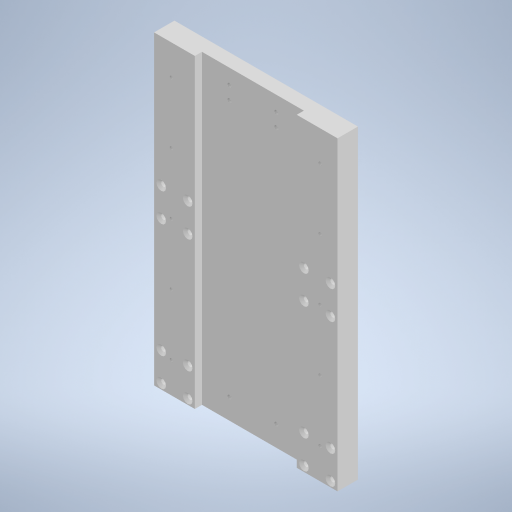
# Autodesk Inventor part: KreuzplatteNeu
Saved by Autodesk Inventor 2024 (Build 280153020, 153B)
## iProperties
Created: 2023-07-13
Part Number: KreuzplatteNeu
Material: Generisch
Document SubType Name: Modeling
Designer: hol
Density: 1 g/cm^3
Appearance: Vorgabe
Author: hol
Autodesk Inventor part; units mm, degrees
ref_plane "YZ Plane" through (0, 0, 0) normal (1, 0, 0) x (0, 1, 0)
ref_plane "XZ Plane" through (0, 0, 0) normal (0, 1, 0) x (-1, 0, 0)
ref_plane "XY Plane" through (0, 0, 0) normal (0, 0, 1) x (1, 0, 0)
sketch "Skizze1" plane through (0, 0, 0) normal (0, 1, 0) x (-1, 0, 0)
  line L0 (0, 0) -> (180, 0)
  line L1 (180, 0) -> (180, 300)
  line L2 (180, 300) -> (0, 300)
  line L3 (0, 300) -> (0, 0)
  dimension "Breite" = 180
  dimension "Höhe" = 300
  constraints: 8 end point, 2 parallel, 1 horizontal, 1 perpendicular
  measures "Breite" distance of L2.end L1.end
  measures "Höhe" distance of L1.end L0.end
extrude "Extrusion1" add sketch "Skizze1" along normal blind 20
sketch "Skizze2" plane through (0, 0, 0) normal (0, -1, 0) x (1, 0, 0)
  line L0 (-180, 300) -> (0, 300) projected
  line L1 (0, 300) -> (0, 0) projected
  line L2 (0, 0) -> (-180, 0) projected
  line L3 (-140, 300) -> (-40, 300)
  line L4 (-40, 300) -> (-40, 0)
  line L5 (-40, 0) -> (-140, 0)
  line L6 (-140, 0) -> (-140, 300)
  point P0 (-90, 300)
  point P1 (-140, 0)
  point P2 (-40, 300)
  dimension "d4" = 100
  constraints: 8 end point, 2 midpoint, 2 parallel, 2 point on line, 1 horizontal, 1 perpendicular
  measures "d4" distance of L3.start L3.end
extrude "Extrusion2" cut sketch "Skizze2" against normal blind 7 contours L0 L4 L2 L6
sketch "Skizze3" plane through (0, 0, 0) normal (0, -1, 0) x (1, 0, 0)
  line L0 (-180, 0) -> (-180, 300) projected
  line L1 (-140, 0) -> (-180, 0) projected
  line L2 (-40, 0) -> (-140, 0) projected
  line L3 (-173, 33.5) -> (-147, 33.5) construction
  line L4 (-147, 33.5) -> (-147, 5.5) construction
  line L5 (-147, 5.5) -> (-173, 5.5) construction
  line L6 (-173, 5.5) -> (-173, 33.5) construction
  point P0 (0, 0)
  dimension "SenkerY" = 26
  dimension "SenkerZ" = 28
  dimension "d9" = 7
  dimension "d10" = 5.5
  constraints: 8 end point, 4 coincident, 2 parallel, 1 horizontal, 1 perpendicular
  measures "SenkerY" distance of L3.start L3.end
  measures "SenkerZ" distance of L5.end L3.start
  measures "d9" distance from line of L0 L5.end
  measures "d10" distance between parallel lines of L1 L5
hole "Bohrung1" at (-173, 0, 5.5) at (-173, 0, 33.5) at (-147, 0, 33.5) at (-147, 0, 5.5) direction (0, 1, 0) diameter 4.8 depth 20 tip angle 118 countersink diameter 9.4 countersink angle 90 clearance for "Flachkopfsenkschraube ISO 2009/7046" size "M4" standard "ISO"
pattern_linear "Rechteckige Anordnung1" count 2 spacing 140 along (0, 0, 1) count 2 spacing 140 along (1, 0, 0) of "Bohrung1"
sketch "Skizze4" plane through (0, 0, 0) normal (0, -1, 0) x (1, 0, 0)
  line L0 (-180, 0) -> (-180, 300) projected
  line L1 (-180, 300) -> (0, 300) construction
  line L2 (-140, 0) -> (-180, 0) construction
  point P0 (0, 0)
  point P1 (-163, 30)
  point P2 (-160, 0)
  dimension "d25" = 30
  dimension "GleitschieneY" = 17
  constraints: 1 midpoint
  measures "d25" vertical distance of point (-160, 0) point (-163, 30)
  measures "GleitschieneY" distance from line of L0 point (-163, 30)
hole "Bohrung2" at (-163, 0, 30) direction (0, 1, 0) diameter 3.242 depth 20 tip angle 118 thread size "M4x0.7" class "6H" standard "ISO Metric profile"
pattern_linear "Rechteckige Anordnung2" count 5 spacing 60 along (0, 0, 1) count 2 spacing 146 along (1, 0, 0) of "Bohrung2"
sketch "Skizze5" plane through (0, 7, 0) normal (0, -1, 0) x (1, 0, 0)
  line L0 (-180, 300) -> (0, 300) construction
  line L1 (-90, 300) -> (-90, 0) construction
  line L2 (-140, 300) -> (-40, 300) construction
  line L3 (-113, 285) -> (-67, 285) construction
  line L4 (-113, 272) -> (-67, 272) construction
  line L5 (-113, 20) -> (-67, 20) construction
  point P0 (0, 0)
  point P1 (-90, 285)
  point P2 (-90, 272)
  point P3 (-90, 20)
  dimension "d40" = 46
  dimension "d41" = 46
  dimension "d42" = 15
  dimension "d43" = 13
  dimension "d44" = 46
  dimension "d45" = 265
  constraints: 8 coincident, 8 end point, 7 midpoint, 3 horizontal, 2 point on line, 1 vertical, 1 vertical alignment
  measures "d40" distance of L3.end L3.start
  measures "d41" distance of L4.end L4.start
  measures "d42" distance from line of L0 point (-90, 285)
  measures "d43" distance from line of point (-90, 285) L4
  measures "d44" distance of L5.end L5.start
  measures "d45" distance of point (-90, 285) point (-90, 20)
hole "Bohrung3" at (-113, 7, 285) at (-67, 7, 285) at (-67, 7, 272) at (-113, 7, 272) at (-113, 7, 20) at (-67, 7, 20) direction (0, 1, 0) diameter 4.134 depth 13 tip angle 118 thread size "M5x0.8" class "6H" standard "ISO Metric profile"
equation "\"d9\" = SenkerYVersatz"
equation "\"d10\" = SenkerZVersatz"
equation "\"d20\" = SenkerPatZ"
equation "\"d23\" = SenkerPatY"
equation "\"d39\" = Breite - 2 * GleitschieneY"
equation "\"SenkerZVersatz\" = 5.5"
equation "\"SenkerYVersatz\" = 7"
equation "\"SenkerPatY\" = -SenkerY + Breite - 2 * SenkerYVersatz"
equation "\"SenkerPatZ\" = 140"
